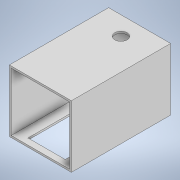
# Autodesk Inventor part: bloc station
Saved by Autodesk Inventor 2020.2 (Build 242310000, 310)
## iProperties
Created: 2020-01-21
Part Number: bloc station
Material: Générique
Document SubType Name: Modeling
Designer: anton
Density: 1 g/cm^3
Appearance: Par défaut
Author: anton
Autodesk Inventor part; units mm, degrees
ref_plane "YZ Plane" through (0, 0, 0) normal (1, 0, 0) x (0, 1, 0)
ref_plane "XZ Plane" through (0, 0, 0) normal (0, 1, 0) x (-1, 0, 0)
ref_plane "XY Plane" through (0, 0, 0) normal (0, 0, 1) x (1, 0, 0)
sketch "Esquisse2" plane through (0, 0, 0) normal (0, 0, 1) x (1, 0, 0)
  line L0 (-49.9248, 43.0827) -> (50.0752, 43.0827)
  line L1 (50.0752, 43.0827) -> (50.0752, -56.9173)
  line L2 (50.0752, -56.9173) -> (-49.9248, -56.9173)
  line L3 (-49.9248, -56.9173) -> (-49.9248, 43.0827)
  point P0 (0, 0)
  dimension "d0" = 100
  dimension "d1" = 100
  constraints: 8 end point, 2 parallel, 1 horizontal, 1 perpendicular
  measures "d0" distance of L0.start L0.end
  measures "d1" distance of L2.end L0.start
extrude "Extrusion1" add sketch "Esquisse2" along normal blind 160
sketch "Esquisse3" plane through (0, 0, 160) normal (0, 0, 1) x (1, 0, 0)
  line L0 (-46.9248, 40.0827) -> (47.0752, 40.0827)
  line L1 (47.0752, 40.0827) -> (47.0752, -53.9173)
  line L2 (47.0752, -53.9173) -> (-46.9248, -53.9173)
  line L3 (-46.9248, -53.9173) -> (-46.9248, 40.0827)
  line L4 (50.0752, 43.0827) -> (-49.9248, 43.0827) projected
  line L5 (50.0752, -56.9173) -> (50.0752, 43.0827) projected
  line L6 (-49.9248, -56.9173) -> (50.0752, -56.9173) projected
  line L7 (-49.9248, 43.0827) -> (-49.9248, -56.9173) projected
  point P0 (0, 0)
  dimension "d4" = 3
  dimension "d5" = 3
  dimension "d6" = 3
  dimension "d7" = 3
  constraints: 8 end point, 2 parallel, 1 horizontal, 1 perpendicular
  measures "d4" distance between parallel lines of L4 L0
  measures "d5" distance between parallel lines of L5 L1
  measures "d6" distance between parallel lines of L6 L2
  measures "d7" distance between parallel lines of L7 L3
extrude "Extrusion2" cut sketch "Esquisse3" against normal blind 155 contours L0 L1 L2 L3
sketch "Esquisse4" plane through (-49.9248, 43.0827, 0) normal (0, 1, 0) x (1, 0, 0)
  circle A0 centre (50, -30) radius 9.7582
  line L0 (100, 0) -> (100, -160) projected
  line L1 (100, 0) -> (0, 0) projected
  point P0 (49.9248, 0)
  dimension "d10" = 50
  dimension "d11" = 30
  constraints: 1 centre point
  measures "d10" distance from line of L0 A0.centre
  measures "d11" distance from line of L1 A0.centre
hole "Perçage1" at (0.0752, 43.0827, 30) direction (0, -1, 0) diameter 20 depth 8 tip angle 118
sketch "Esquisse5" plane through (-49.9248, -56.9173, 0) normal (0, -1, 0) x (1, 0, 0)
  line L0 (20, 150) -> (80, 150)
  line L1 (80, 150) -> (80, 30)
  line L2 (80, 30) -> (20, 30)
  line L3 (20, 30) -> (20, 150)
  line L4 (0, 0) -> (100, 0) projected
  line L5 (100, 0) -> (100, 160) projected
  point P0 (49.9248, 0)
  dimension "d19" = 60
  dimension "d20" = 120
  dimension "d21" = 30
  dimension "d22" = 20
  constraints: 8 end point, 2 parallel, 1 horizontal, 1 perpendicular
  measures "d19" distance of L0.start L0.end
  measures "d20" distance of L0.end L1.end
  measures "d21" distance between parallel lines of L4 L2
  measures "d22" distance between parallel lines of L5 L1
extrude "Extrusion3" cut sketch "Esquisse5" against normal blind 5
